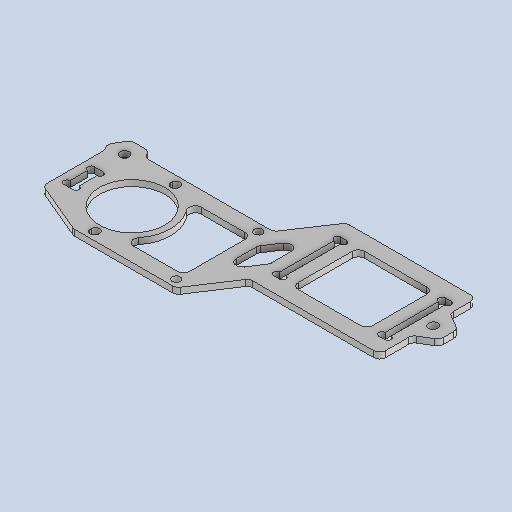
# Autodesk Inventor part: Ankle_side_frame
Saved by Autodesk Inventor 2022.4 (Build 264492000, 492)
## iProperties
Created: 2021-10-01
Part Number: Ankle_side_frame
Material: アルミニウム 2014-T4
Document SubType Name: Modeling
Designer: Masato Kubotera
Density: 2.8 g/cm^3
Appearance: 滑らか - 淡い灰色
Description: A2017 T2
Mass: 9.96642 g
Surface Area: 50.588 cm^2
Volume: 3.55944 cm^3
Author: Masato Kubotera
Autodesk Inventor part; units mm, degrees
ref_plane "YZ Plane" through (0, 0, 0) normal (1, 0, 0) x (0, 1, 0)
ref_plane "XZ Plane" through (0, 0, 0) normal (0, 1, 0) x (-1, 0, 0)
ref_plane "XY Plane" through (0, 0, 0) normal (0, 0, 1) x (1, 0, 0)
sketch "スケッチ1" plane through (0, 0, 0) normal (0, 0, 1) x (1, 0, 0)
  line L0 (28, 13.5) -> (1, 13.5) construction
  line L1 (1, 13.5) -> (1, -13.5) construction
  line L2 (1, -13.5) -> (28, -13.5) construction
  line L3 (28, -13.5) -> (28, 13.5) construction
  line L4 (28, 13.5) -> (1, -13.5) construction
  line L5 (1, 13.5) -> (28, -13.5) construction
  circle A0 centre (0, 0) radius 10.5 construction
  circle A1 centre (0, 0) radius 10.75
  arc A2 (0, 16) -> (-12, 10.583) centre (0, 0) ccw construction
  line L6 (1, 0) -> (28, 0) construction
  line L7 (14.5, 13.5) -> (14.5, -13.5) construction
  circle A3 centre (28, 13.5) radius 1.35
  arc A4 (-0.35, 13) -> (2.35, 13) centre (1, 13) ccw
  line L8 (2.35, 13.5) -> (2.35, 13)
  line L9 (-0.35, 13.5) -> (-0.35, 13)
  arc A5 (2.35, 13.5) -> (-0.35, 13.5) centre (1, 13.5) ccw
  line L10 (-12, 10.583) -> (-12, -10.583) construction
  arc A6 (-12, -10.583) -> (0, -16) centre (0, 0) ccw construction
  circle A7 centre (28, -13.5) radius 1.35
  arc A8 (2.35, -13) -> (-0.35, -13) centre (1, -13) ccw
  line L11 (2.35, -13.5) -> (2.35, -13)
  line L12 (-0.35, -13.5) -> (-0.35, -13)
  arc A9 (-0.35, -13.5) -> (2.35, -13.5) centre (1, -13.5) ccw
  line L13 (-17.5, 5) -> (-14.5, 5) construction
  line L14 (-14.5, 5) -> (-14.5, -5) construction
  line L15 (-14.5, -5) -> (-17.5, -5) construction
  line L16 (-17.5, -5) -> (-17.5, 5) construction
  line L17 (-17.5, 5) -> (-14.5, -5) construction
  line L18 (-14.5, 5) -> (-17.5, -5) construction
  line L19 (-17.51, 5.01) -> (-14.49, 5.01)
  line L20 (-14.49, 5.01) -> (-14.49, 2.91) construction
  line L21 (-14.49, -5.01) -> (-17.51, -5.01)
  line L22 (-17.51, -5.01) -> (-17.51, -2.91) construction
  line L23 (-17.51, 5.01) -> (-14.49, -5.01) construction
  line L24 (-14.49, 5.01) -> (-17.51, -5.01) construction
  arc A10 (-17.51, 5.01) -> (-17.51, 2.91) centre (-17.51, 3.96) ccw
  line L25 (-17.5, 0) -> (-14.5, 0) construction
  line L26 (-16, 5) -> (-16, -5) construction
  arc A11 (-14.49, 2.91) -> (-14.49, 5.01) centre (-14.49, 3.96) ccw
  arc A12 (-17.51, -2.91) -> (-17.51, -5.01) centre (-17.51, -3.96) ccw
  arc A13 (-14.49, -5.01) -> (-14.49, -2.91) centre (-14.49, -3.96) ccw
  line L27 (-17.51, 2.91) -> (-17.51, 5.01) construction
  line L28 (-17.51, -2.91) -> (-17.51, 2.91)
  line L29 (-14.49, -2.91) -> (-14.49, -5.01) construction
  line L30 (-14.49, 2.91) -> (-14.49, -2.91)
  circle A14 centre (-16, 13.5) radius 1.55
  line L31 (-20.5, 11.2942) -> (-20.5, -8.739)
  line L32 (-20.5, -8.739) -> (-3.2261, -16)
  line L33 (-3.2261, -16) -> (30.4, -16)
  line L34 (-11.6699, 16) -> (30.4, 16)
  arc A15 (6.2732, -11.1) -> (6.2732, 11.1) centre (0, 0) ccw
  line L35 (6.2732, 11.1) -> (28, 11.1)
  circle A16 centre (28, 13.5) radius 2.4 construction
  circle A17 centre (28, -13.5) radius 2.4 construction
  line L36 (6.2732, -11.1) -> (28, -11.1)
  line L37 (79.5, 25.4) -> (77.5, 25.4) construction
  line L38 (77.5, 25.4) -> (77.5, 3.6) construction
  line L39 (77.5, 3.6) -> (79.5, 3.6) construction
  line L40 (79.5, 3.6) -> (79.5, 25.4) construction
  line L41 (79.5, 25.4) -> (77.5, 3.6) construction
  line L42 (77.5, 25.4) -> (79.5, 3.6) construction
  line L43 (77.49, 25.41) -> (79.51, 25.41)
  line L44 (79.51, 25.41) -> (79.51, 23.31) construction
  line L45 (79.51, 3.59) -> (77.49, 3.59)
  line L46 (77.49, 3.59) -> (77.49, 5.69) construction
  line L47 (77.49, 25.41) -> (79.51, 3.59) construction
  line L48 (79.51, 25.41) -> (77.49, 3.59) construction
  arc A18 (77.49, 25.41) -> (77.49, 23.31) centre (77.49, 24.36) ccw
  line L49 (78.5, 25.4) -> (78.5, 3.6) construction
  line L50 (77.5, 14.5) -> (79.5, 14.5) construction
  arc A19 (79.51, 23.31) -> (79.51, 25.41) centre (79.51, 24.36) ccw
  arc A20 (77.49, 5.69) -> (77.49, 3.59) centre (77.49, 4.64) ccw
  arc A21 (79.51, 3.59) -> (79.51, 5.69) centre (79.51, 4.64) ccw
  line L51 (77.49, 23.31) -> (77.49, 25.41) construction
  line L52 (79.51, 23.31) -> (79.51, 5.69)
  line L53 (79.51, 5.69) -> (79.51, 3.59) construction
  line L54 (77.49, 5.69) -> (77.49, 23.31)
  circle A22 centre (83.5, 15.5) radius 1.55
  line L55 (83.5, 12.0359) -> (80.5, 13.7679) construction
  line L56 (80.5, 13.7679) -> (80.5, 17.2321) construction
  line L57 (80.5, 17.2321) -> (83.5, 18.9641) construction
  line L58 (83.5, 18.9641) -> (86.5, 17.2321) construction
  line L59 (86.5, 17.2321) -> (86.5, 13.7679) construction
  line L60 (86.5, 13.7679) -> (83.5, 12.0359) construction
  line L61 (40, 30.4) -> (82.75, 30.4)
  line L62 (82.75, 30.4) -> (82.75, 21.7065)
  line L63 (82.75, 21.7065) -> (88.5, 18.3868)
  line L64 (88.5, 18.3868) -> (88.5, 12.6132)
  line L65 (88.5, 12.6132) -> (82.75, 9.2935)
  line L66 (82.75, 9.2935) -> (82.75, -1.4)
  line L67 (82.75, -1.4) -> (40, -1.4)
  line L68 (30.4, -16) -> (40, -1.4)
  line L69 (40, 30.4) -> (40, -1.4) construction
  line L70 (32, 9.3861) -> (32, -4.4659)
  line L71 (32, -4.4659) -> (39, 6.1799)
  line L72 (39, 6.1799) -> (39, 19.8861)
  line L73 (39, 19.8861) -> (32, 9.3861)
  line L74 (-17.5, 10) -> (-14.5, 10) construction
  line L75 (-14.5, -10) -> (-17.5, -10) construction
  line L76 (-17.5, 10) -> (-14.5, -10) construction
  line L77 (-14.5, 10) -> (-17.5, -10) construction
  line L78 (40, 30.4) -> (30.4, 16)
  line L79 (30.4, 16) -> (30.4, -16) construction
  line L80 (43, 25.5) -> (45, 25.5) construction
  line L81 (45, 25.5) -> (45, 3.5) construction
  line L82 (45, 3.5) -> (43, 3.5) construction
  line L83 (43, 3.5) -> (43, 25.5) construction
  line L84 (43, 25.5) -> (45, 3.5) construction
  line L85 (45, 25.5) -> (43, 3.5) construction
  line L86 (42.99, 25.51) -> (45.01, 25.51)
  line L87 (45.01, 25.51) -> (45.01, 23.41)
  line L88 (45.01, 3.49) -> (42.99, 3.49)
  line L89 (42.99, 3.49) -> (42.99, 5.59) construction
  line L90 (42.99, 25.51) -> (45.01, 3.49) construction
  line L91 (45.01, 25.51) -> (42.99, 3.49) construction
  line L92 (44, 25.5) -> (44, 3.5) construction
  line L93 (43, 14.5) -> (45, 14.5) construction
  arc A23 (42.99, 25.51) -> (42.99, 23.41) centre (42.99, 24.46) ccw
  arc A24 (45.01, 23.41) -> (45.01, 25.51) centre (45.01, 24.46) ccw
  arc A25 (42.99, 5.59) -> (42.99, 3.49) centre (42.99, 4.54) ccw
  arc A26 (45.01, 3.49) -> (45.01, 5.59) centre (45.01, 4.54) ccw
  line L94 (45.01, 23.41) -> (45.01, 5.59)
  line L95 (42.99, 5.59) -> (42.99, 25.51)
  line L96 (45.01, 5.59) -> (45.01, 3.49) construction
  line L97 (28, 11.1) -> (28, -11.1)
  line L98 (49, 25.4) -> (49, 3.6)
  line L99 (49, 3.6) -> (73.5, 3.6)
  line L100 (73.5, 3.6) -> (73.5, 25.4)
  line L101 (73.5, 25.4) -> (49, 25.4)
  line L102 (-17.7321, 10.5) -> (-19.4641, 13.5) construction
  line L103 (-19.4641, 13.5) -> (-17.7321, 16.5) construction
  line L104 (-17.7321, 16.5) -> (-14.2679, 16.5) construction
  line L105 (-14.2679, 16.5) -> (-12.5359, 13.5) construction
  line L106 (-12.5359, 13.5) -> (-14.2679, 10.5) construction
  line L107 (-14.2679, 10.5) -> (-17.7321, 10.5) construction
  line L108 (-20.5, 11.2942) -> (-21.7735, 13.5)
  line L109 (-21.7735, 13.5) -> (-18.8868, 18.5)
  line L110 (-18.8868, 18.5) -> (-13.1132, 18.5)
  line L111 (-13.1132, 18.5) -> (-11.6699, 16)
  point P0 (14.5, 0)
  point P1 (-16, 0)
  point P2 (-16, 0)
  point P3 (78.5, 14.5)
  point P4 (44, 14.5)
  dimension "d0" = 27
  dimension "d1" = 27
  dimension "d2" = 21
  dimension "d3" = 0.25
  dimension "d6" = 2.7
  dimension "d9" = 0.5
  dimension "d10" = 1.35
  dimension "d11" = 1
  dimension "d12" = 16
  dimension "d13" = 12
  dimension "d14" = 3
  dimension "d16" = 2.5
  dimension "d18" = 0.01
  dimension "d20" = 3.1
  dimension "d28" = 3
  dimension "d29" = 4.8
  dimension "d52" = 2
  dimension "d53" = 4.8
  dimension "d54" = 10
  dimension "d55" = 0.01
  dimension "d56" = 1.05
  dimension "d75" = 1.05
  dimension "d76" = 0.01
  dimension "d77" = 0.01
  dimension "d80" = 3.1
  dimension "d86" = 3.25
  dimension "d87" = 2
  dimension "d88" = 2
  dimension "d89" = 5
  dimension "d90" = 2
  dimension "d91" = 6
  dimension "d92" = 2
  dimension "d93" = 5
  dimension "d95" = 1
  dimension "d96" = 5
  dimension "d97" = 21.8
  dimension "d104" = 5
  dimension "d109" = 5
  dimension "d110" = 5
  dimension "d111" = 2
  dimension "d112" = 22
  dimension "d113" = 1.05
  dimension "d115" = 0.01
  dimension "d116" = 0.01
  dimension "d117" = 32.5
  dimension "d118" = 45
  dimension "d120" = 4
  dimension "d121" = 4
  dimension "d122" = 3
  dimension "d124" = 14.5
  dimension "d125" = 5
  dimension "d126" = 5
  dimension "d127" = 4
  dimension "d128" = 4
  dimension "d129" = 6
  dimension "d130" = 0.5
  dimension "d131" = 2
  dimension "d132" = 2
  dimension "d133" = 2
  dimension "d134" = 2
  dimension "d135" = 17
  dimension "d136" = 20
  constraints: 226 end point, 46 parallel, 38 point on circle, 35 midpoint, 28 symmetric about line, 27 centre point, 20 perpendicular, 16 point on line, 12 horizontal, 11 coincident, 8 tangent, 6 vertical, 3 collinear, 39 other
  measures "d0" distance of L2.end L1.end
  measures "d1" distance of L1.end L0.end
  measures "d2" diameter of A0
  measures "d3" radial gap between concentric circles of A1 A0
  measures "d6" diameter of A3
  measures "d9" distance of A4.centre L0.end
  measures "d10" radius of A5
  measures "d11" distance of point (0, 0) L6.start
  measures "d12" radius of A2
  measures "d13" distance from line of L10 A0.centre
  measures "d14" distance of L14.end L15.end
  measures "d16" distance between parallel lines of L10 L14
  measures "d18" distance between parallel lines of L19 L13
  measures "d20" diameter of A14
  measures "d28" distance between parallel lines of L31 L16
  measures "d29" diameter of A16
  measures "d52" radial gap between concentric circles of A1 A15
  measures "d53" diameter of A17
  measures "d54" distance between parallel lines of L15 L13
  measures "d55" distance between parallel lines of L16 L27
  measures "d56" radius of A10
  measures "d75" radius of A18
  measures "d76" distance between parallel lines of L37 L43
  measures "d77" distance between parallel lines of L46 L38
  measures "d80" diameter of A22
  measures "d86" distance between parallel lines of L62 L40
  measures "d87" distance between parallel lines of L64 L59
  measures "d88" distance between parallel lines of L63 L58
  measures "d89" horizontal distance of point (83.5, 15.5) point (78.5, 14.5)
  measures "d90" distance between parallel lines of L65 L60
  measures "d91" distance between parallel lines of L60 L57
  measures "d92" distance between parallel lines of L38 L40
  measures "d93" distance between parallel lines of L61 L37
  measures "d95" vertical distance of point (78.5, 14.5) A22.centre
  measures "d96" distance between parallel lines of L67 L39
  measures "d97" distance between parallel lines of L39 L37
  measures "d104" distance between parallel lines of L68 L71
  measures "d109" distance between parallel lines of L13 L74
  measures "d110" distance between parallel lines of L78 L73
  measures "d111" distance of L81.end L82.end
  measures "d112" distance of L80.end L81.end
  measures "d113" radius of A23
  measures "d115" distance between parallel lines of L86 L80
  measures "d116" distance between parallel lines of L89 L83
  measures "d117" distance between parallel lines of L38 L81
  measures "d118" distance from line of L81 point (0, 0)
  measures "d120" distance between parallel lines of L97 L70
  measures "d121" distance between parallel lines of L83 L72
  measures "d122" distance between parallel lines of L69 L83
  measures "d124" distance between parallel lines of L6 L93
  measures "d125" distance between parallel lines of L101 L61
  measures "d126" distance between parallel lines of L67 L99
  measures "d127" distance between parallel lines of L81 L98
  measures "d128" distance between parallel lines of L100 L38
  measures "d129" distance between parallel lines of L102 L105
  measures "d130" distance between parallel lines of L107 L74
  measures "d131" distance between parallel lines of L109 L103
  measures "d132" distance between parallel lines of L110 L104
  measures "d133" distance between parallel lines of L108 L102
  measures "d134" distance between parallel lines of L111 L105
  measures "d135" distance from line of point (-16, 13.5) L1
  measures "d136" distance between parallel lines of L75 L74
extrude "押し出し1" add sketch "スケッチ1" along normal blind 2
fillet "フィレット1" radius 2 17 edges at (-20.5, 11.2942, 1) (-20.5, -8.739, 1) (-3.2261, -16, 1) (30.4, 16, 1) (40, 30.4, 1) (82.75, 30.4, 1) (82.75, 21.7065, 1) (88.5, 18.3868, 1) (88.5, 12.6132, 1) (82.75, 9.2935, 1) (82.75, -1.4, 1) (40, -1.4, 1) (30.4, -16, 1) (-21.7735, 13.5, 1) (-18.8868, 18.5, 1) (-13.1132, 18.5, 1) (-11.6699, 16, 1)
fillet "フィレット2" radius 2 12 edges at (6.2732, 11.1, 1) (6.2732, -11.1, 1) (32, 9.3861, 1) (32, -4.4659, 1) (39, 6.1799, 1) (39, 19.8861, 1) (28, -11.1, 1) (28, 11.1, 1) (49, 25.4, 1) (49, 3.6, 1) (73.5, 3.6, 1) (73.5, 25.4, 1)
equation "\"d10\" = 0.5 * d6"
